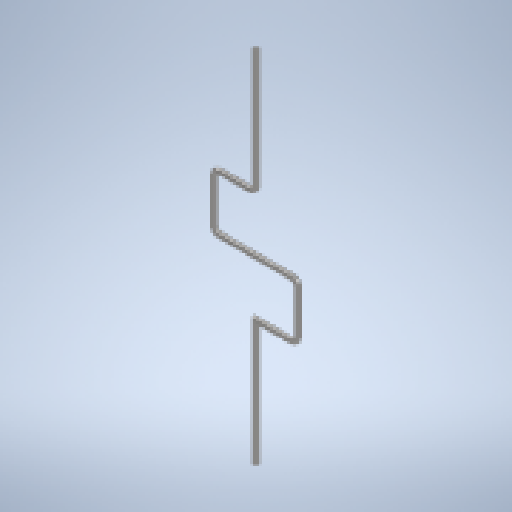
# Autodesk Inventor part: Trittstange
Saved by Autodesk Inventor 2024.4 (Build 284460000, 460)
## iProperties
Created: 2026-01-10
Part Number: Trittstange
Material: Edelstahl
Description: Trittstange
Document SubType Name: Modeling
Designer: Philf
Mass: 4742.75 g
Surface Area: 1191.97 cm^2
Volume: 592.844 cm^3
Density: 8 g/cm^3
Appearance: Halbpoliert
Masse[kg]: 3,411 kg
durchmesser: 20,000 mm
Autodesk Inventor part; units mm, degrees
ref_plane "YZ Plane" through (0, 0, 0) normal (1, 0, 0) x (0, 1, 0)
ref_plane "XZ Plane" through (0, 0, 0) normal (0, 1, 0) x (-1, 0, 0)
ref_plane "XY Plane" through (0, 0, 0) normal (0, 0, 1) x (1, 0, 0)
sketch "Skizze1" plane through (0, 0, 0) normal (0, 1, 0) x (-1, 0, 0)
  line L0 (0, 0) -> (0, -445)
  line L1 (20, -465) -> (130, -465)
  line L2 (150, -485) -> (150, -645)
  line L3 (130, -665) -> (-130, -665)
  line L4 (-150, -685) -> (-150, -845)
  line L5 (-130, -865) -> (0, -865)
  line L6 (0, -865) -> (0, -1330)
  arc A0 (150, -485) -> (130, -465) centre (130, -485) ccw
  arc A1 (130, -665) -> (150, -645) centre (130, -645) ccw
  arc A2 (0, -445) -> (20, -465) centre (20, -445) ccw
  arc A3 (-130, -665) -> (-150, -685) centre (-130, -685) ccw
  arc A4 (-150, -845) -> (-130, -865) centre (-130, -845) ccw
  point P0 (0, -465)
  point P1 (150, -465)
  point P2 (150, -665)
  point P3 (-150, -665)
  point P4 (-150, -865)
  dimension "lange1" = 465
  dimension "d1" = 150
  dimension "d2" = 200
  dimension "d3" = 300
  dimension "d4" = 200
  dimension "lange2" = 465
  dimension "d6" = 20
  constraints: 14 end point, 10 point on circle, 10 point on line, 10 tangent, 5 centre point, 5 perpendicular, 4 equal radius, 1 horizontal, 1 vertical
  measures "lange1" distance of L0.start point (0, -465)
  measures "d1" distance of point (0, -465) point (150, -465)
  measures "d2" distance of point (150, -465) point (150, -665)
  measures "d3" distance of point (150, -665) point (-150, -665)
  measures "d4" distance of point (-150, -665) point (-150, -865)
  measures "lange2" distance of L5.end L6.end
  measures "d6" radius of A0
sketch "Skizze2" plane through (0, 0, 0) normal (0, 0, 1) x (1, 0, 0)
  circle A0 centre (0, 0) radius 10
  dimension "durchmesser" = 20
  constraints: 1 centre point, 1 coincident
  measures "durchmesser" diameter of A0
sweep "Sweeping1" add profiles "Skizze2" path "Skizze1"
